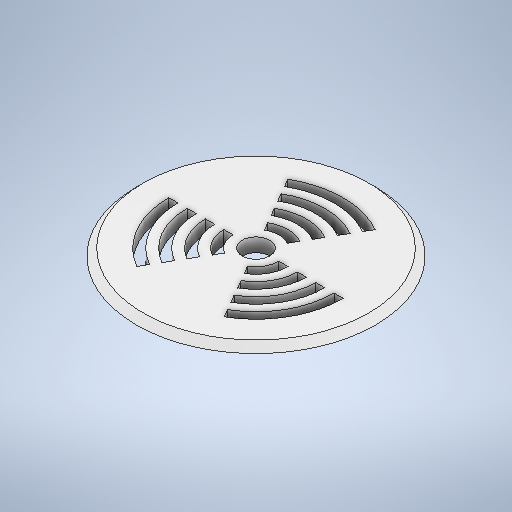
# Autodesk Inventor part: cover
Saved by Autodesk Inventor 2025.2 (Build 292293000, 293)
## iProperties
Created: 2025-03-24
Part Number: cover
Material: LCP plast
Document SubType Name: Modeling
Designer: hepma_axt67em
Density: 1.626 g/cm^3
Appearance: Hladká – bílá
Mass: 7.54649 g
Surface Area: 50.301 cm^2
Volume: 4.64114 cm^3
Author: hepma_axt67em
Autodesk Inventor part; units mm, degrees
ref_plane "YZ Plane" through (0, 0, 0) normal (1, 0, 0) x (0, 1, 0)
ref_plane "XZ Plane" through (0, 0, 0) normal (0, 1, 0) x (-1, 0, 0)
ref_plane "XY Plane" through (0, 0, 0) normal (0, 0, 1) x (1, 0, 0)
sketch "Náčrt1" plane through (0, 0, 0) normal (0, 1, 0) x (-1, 0, 0)
  line L0 (0, -38.2576) -> (0, 38.2576) projected
  line L1 (-38.2576, 0) -> (38.2576, 0) projected
  circle A0 centre (0, 0) radius 23.55
  dimension "d0" = 47.1
  constraints: 1 centre point, 1 coincident
  measures "d0" diameter of A0
extrude "Vysunutí1" add sketch "Náčrt1" along normal blind 1.5
sketch "Náčrt2" plane through (0, 1.5, 0) normal (0, 1, 0) x (1, 0, 0)
  line L0 (0, 36.47) -> (0, -36.47) projected
  line L1 (36.47, 0) -> (-36.47, 0) projected
  circle A0 centre (0, 0) radius 26.05
  dimension "d3" = 52.1
  constraints: 1 centre point, 1 coincident
  measures "d3" diameter of A0
extrude "Vysunutí2" add sketch "Náčrt2" along normal blind 1.5
chamfer "Zkosení1" distance 1.5 angle 45 1 edges at (-26.05, 3, 0)
sketch "Náčrt3" plane through (0, 3, 0) normal (0, 1, 0) x (1, 0, 0)
  line L0 (0, 36.47) -> (0, -36.47) projected
  line L1 (36.47, 0) -> (-36.47, 0) projected
  arc A0 (2.5, 4.3301) -> (-2.5, 4.3301) centre (0, 0) ccw
  arc A1 (3.5, 6.0622) -> (-3.5, 6.0622) centre (0, 0) ccw
  line L2 (-2.5, 4.3301) -> (-3.5, 6.0622)
  line L3 (2.5, 4.3301) -> (3.5, 6.0622)
  arc A2 (4.5, 7.7942) -> (-4.5, 7.7942) centre (0, 0) ccw
  arc A3 (5.5, 9.5263) -> (-5.5, 9.5263) centre (0, 0) ccw
  line L4 (-4.5, 7.7942) -> (-5.5, 9.5263)
  line L5 (4.5, 7.7942) -> (5.5, 9.5263)
  arc A4 (6.5, 11.2583) -> (-6.5, 11.2583) centre (0, 0) ccw
  arc A5 (7.5, 12.9904) -> (-7.5, 12.9904) centre (0, 0) ccw
  line L6 (-6.5, 11.2583) -> (-7.5, 12.9904)
  line L7 (6.5, 11.2583) -> (7.5, 12.9904)
  arc A6 (8.5, 14.7224) -> (-8.5, 14.7224) centre (0, 0) ccw
  arc A7 (9.5, 16.4545) -> (-9.5, 16.4545) centre (0, 0) ccw
  line L8 (-8.5, 14.7224) -> (-9.5, 16.4545)
  line L9 (8.5, 14.7224) -> (9.5, 16.4545)
  dimension "d10" = 5
  dimension "d11" = 7
  dimension "d12" = 60
  dimension "d24" = 9
  dimension "d25" = 11
  dimension "d26" = 13
  dimension "d27" = 15
  dimension "d28" = 17
  dimension "d29" = 19
  constraints: 16 end point, 16 point on circle, 8 centre point, 7 coincident, 6 collinear, 2 midpoint, 1 point on line, 1 other
  measures "d10" radius of A0
  measures "d11" radius of A1
  measures "d12" angle of L3 L2
  measures "d24" radius of A2
  measures "d25" radius of A3
  measures "d26" radius of A4
  measures "d27" radius of A5
  measures "d28" radius of A6
  measures "d29" radius of A7
extrude "Vysunutí3" cut sketch "Náčrt3" against normal through all
pattern_circular "Kruhové pole1" count 3 over 360 about axis through (0, -10, 0) along (0, 1, 0) of "Vysunutí3"
sketch "Náčrt4" plane through (0, 3, 0) normal (0, 1, 0) x (1, 0, 0)
  line L0 (0, 36.47) -> (0, -36.47) projected
  line L1 (36.47, 0) -> (-36.47, 0) projected
  circle A0 centre (0, 0) radius 3
  dimension "d18" = 6
  constraints: 1 centre point, 1 coincident
  measures "d18" diameter of A0
extrude "Vysunutí4" cut sketch "Náčrt4" against normal through all
